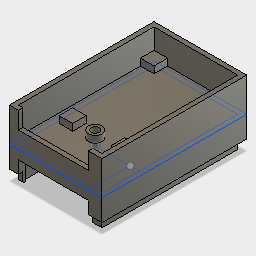
esp-dsc-v1-case (Autodesk Fusion 360 design; units mm, degrees)
Autodesk Fusion 360 part; units mm, degrees
sketch "Sketch1" plane through (0, 0, 0) normal (0, 1, 0) x (1, 0, 0)
  line L0 (-15, 25) -> (22, 25)
  line L1 (22, 25) -> (22, -35)
  line L2 (-15, -35) -> (-15, 25)
  line L3 (-15, -35) -> (-13, -35)
  line L4 (22, -35) -> (18, -35)
  line L5 (24, -37) -> (-17, -37)
  line L6 (-17, -37) -> (-17, 27)
  line L7 (-17, 27) -> (24, 27)
  line L8 (24, 27) -> (24, -37)
  line L9 (18, -35) -> (18, -37)
  line L10 (-13, -35) -> (-13, -37)
  line L11 (18, -35) -> (18, -18.5)
  line L12 (22, -18.5) -> (2.5, -18.5)
  circle A0 centre (2.5, -18.5) radius 1.8
  line L13 (-13, -35) -> (18, -35)
  dimension "d1" = 37
  dimension "d2" = 60
  dimension "d4" = 2
  dimension "d5" = 4
  dimension "d6" = 16.5
  dimension "d7" = 19.5
  dimension "d8" = 3.6
  measures "d1" distance of L0.start L0.end
  measures "d2" distance of L0.start L2.start
  measures "d4" distance of L2.start L3.end
  measures "d5" distance of L1.end L4.end
  measures "d6" distance of L4.end L11.end
  measures "d7" distance of L12.start L12.end
  measures "d8" diameter of A0
extrude "Extrude1" add sketch "Sketch1" along normal blind 3 makes body 1
sketch "Sketch2" plane through (0, 3, 0) normal (0, 1, 0) x (-1, 0, 0)
  circle A0 centre (-2.5, 18.5) radius 1.8
  line L0 (-24, -27) -> (17, -27)
  line L1 (17, -27) -> (17, 37)
  line L2 (17, 37) -> (-24, 37)
  line L3 (-24, 37) -> (-24, -27)
  circle A1 centre (-2.5, 18.5) radius 3
  dimension "d11" = 6
  measures "d11" diameter of A1
extrude "Extrude2" add sketch "Sketch2" along normal blind 3 contours A1 bodies 1
extrude "Extrude3" add sketch "Sketch1" along normal blind 15 contours L0 L1 L2 L3 L4 L5 L6 L7 L8 L9 L10 bodies 1
sketch "Sketch3" plane through (0, 3, 0) normal (0, 1, 0) x (-1, 0, 0)
  line L0 (13, 35) -> (13, 37)
  line L1 (13, 37) -> (-18, 37)
  line L2 (-18, 37) -> (-18, 35)
  line L3 (-18, 35) -> (-22, 35)
  line L4 (-22, 35) -> (-22, -25)
  line L5 (-22, -25) -> (15, -25)
  line L6 (15, -25) -> (15, 35)
  line L7 (15, 35) -> (13, 35)
  circle A0 centre (-2.5, 18.5) radius 3
  line L8 (-12, 15) -> (-18, 15)
  line L9 (-18, 15) -> (-18, 21)
  line L10 (-18, 21) -> (-12, 21)
  line L11 (-12, 21) -> (-12, 15)
  line L12 (11, 15) -> (5, 15)
  line L13 (5, 15) -> (5, 21)
  line L14 (5, 21) -> (11, 21)
  line L15 (11, 21) -> (11, 15)
  line L16 (15, -25) -> (9, -25)
  line L17 (9, -25) -> (9, -19)
  line L18 (9, -19) -> (15, -19)
  line L19 (15, -19) -> (15, -25)
  line L20 (-22, -25) -> (-16, -25)
  line L21 (-16, -25) -> (-16, -19)
  line L22 (-16, -19) -> (-22, -19)
  line L23 (-22, -19) -> (-22, -25)
  dimension "d16" = 6
  dimension "d17" = 6
  dimension "d18" = 6
  dimension "d19" = 6
  dimension "d20" = 6
  dimension "d21" = 6
  measures "d16" distance of L8.start L10.end
  measures "d17" distance of L12.start L14.end
  measures "d18" distance of L5.end L16.end
  measures "d19" distance of L5.end L18.end
  measures "d20" distance of L4.end L20.end
  measures "d21" distance of L4.end L22.end
extrude "Extrude4" add sketch "Sketch3" along normal blind 3 contours L5 L6 L16 L17 L18 L19 | L4 L5 L20 L21 L22 L23 | L8 L9 L10 L11 | L12 L13 L14 L15 bodies 1
extrude "Extrude5" add sketch "Sketch1" along normal blind 7.5 contours L5 L9 L10 L13 bodies 1
cylinder "CylinderPrimitive1" cut diameter 4.5 height 3.2 placed x (1, 0, 0) y (0, 0, -1) z (0, 1, 0) at (2.5, 0, 18.5) bodies 1
extrude "Extrude7" add sketch "Sketch1" against normal blind 4 separate body makes body 2
extrude "Extrude8" add sketch "Sketch1" against normal blind 9.5 contours L0 L1 L2 L3 L4 L5 L6 L7 L8 L9 L10 bodies 2
sketch "Sketch5" plane through (0, -4, 0) normal (0, -1, 0) x (1, 0, 0)
  line L0 (18, 35) -> (18, 37)
  line L1 (18, 37) -> (-13, 37)
  line L2 (-13, 37) -> (-13, 35)
  line L3 (-13, 35) -> (-15, 35)
  line L4 (-15, 35) -> (-15, -25)
  line L5 (-15, -25) -> (22, -25)
  line L6 (22, -25) -> (22, 35)
  line L7 (22, 35) -> (18, 35)
  circle A0 centre (2.5, 18.5) radius 1.8
  line L8 (18, 35) -> (18, 34)
  line L9 (18, 34) -> (21, 34)
  line L10 (-13, 35) -> (-13, 34)
  line L11 (-13, 34) -> (-14, 34)
  line L12 (-14, 34) -> (-14, -24)
  line L13 (22, -25) -> (22, -24)
  line L14 (21, -24) -> (-14, -24)
  line L15 (22, -25) -> (21, -25)
  line L16 (21, -24) -> (21, 34)
extrude "Extrude9" add sketch "Sketch5" along normal blind 10 contours L3 L4 L5 L6 L7 L8 L9 L10 L11 L12 L13 L14 L15 L16 bodies 2
chamfer "Chamfer1" distance 0.5 angle 45 5 edges at (-14, -14, 35) (-15, -14, 5) (3.5, -14, -25) (22, -14, 5) (20, -14, 35) on bodies 2
cylinder "CylinderPrimitive2" add diameter 8 height 4 placed x (1, 0, 0) y (0, 0, 1) z (0, -1, 0) at (2.5, -4, 18.5) bodies 2
cylinder "CylinderPrimitive3" cut diameter 6 height -4 placed x (1, 0, 0) y (0, 0, -1) z (0, 1, 0) at (2.5, 0, 18.5) bodies 2
cylinder "CylinderPrimitive4" cut diameter 3.6 height -8 placed x (1, 0, 0) y (0, 0, -1) z (0, 1, 0) at (2.5, 0, 18.5) bodies 2
named bodies: "Top"
